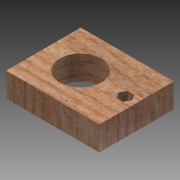
# Autodesk Inventor part: CNC-Z-axis- dremel mount
Saved by Autodesk Inventor 2015 (Build 190159000, 159)
## iProperties
Created: 2015-03-21
Part Number: CNC-Z-axis- dremel mount
Material: Generic
Document SubType Name: Modeling
Designer: Bangladesh
Density: 1 g/cm^3
Appearance: Default
Author: Bangladesh
Autodesk Inventor part; units mm, degrees
ref_plane "YZ Plane" through (0, 0, 0) normal (1, 0, 0) x (0, 1, 0)
ref_plane "XZ Plane" through (0, 0, 0) normal (0, 1, 0) x (-1, 0, 0)
ref_plane "XY Plane" through (0, 0, 0) normal (0, 0, 1) x (1, 0, 0)
sketch "Sketch1" plane through (0, 0, 0) normal (0, 1, 0) x (-1, 0, 0)
  line L0 (50, 40) -> (-50, 40)
  line L1 (-50, 40) -> (-50, -40)
  line L2 (-50, -40) -> (50, -40)
  line L3 (50, -40) -> (50, 40)
  line L4 (50, 40) -> (-50, -40) construction
  line L5 (-50, 40) -> (50, -40) construction
  point P0 (0, 0)
  dimension "d0" = 100
  dimension "d1" = 80
  constraints: 12 end point, 2 midpoint, 2 parallel, 1 horizontal, 1 perpendicular
  measures "d0" distance of L2.end L1.end
  measures "d1" distance of L1.end L0.end
extrude "Extrusion1" add sketch "Sketch1" along normal mid plane 26
sketch "Sketch2" plane through (0, 13, 0) normal (0, 1, 0) x (1, 0, 0)
  circle A0 centre (-10.17, 0) radius 22.33
  line L0 (-50, 40) -> (-50, -40) projected
  circle A1 centre (37.85, 0) radius 7.255
  line L1 (50, -40) -> (50, 40) projected
  line L2 (45.105, 0) -> (41.4775, -6.283)
  line L3 (41.4775, -6.283) -> (34.2225, -6.283)
  line L4 (34.2225, -6.283) -> (30.595, 0)
  line L5 (30.595, 0) -> (34.2225, 6.283)
  line L6 (34.2225, 6.283) -> (41.4775, 6.283)
  line L7 (41.4775, 6.283) -> (45.105, 0)
  dimension "d12" = 14.51
  dimension "d6" = 39.83
  dimension "d8" = 12.15
  constraints: 12 end point, 1 centre point, 1 coincident, 1 horizontal alignment, 15 other
  measures "d6" distance from line of L0 A0.centre
  measures "d8" distance from line of L1 point (37.85, 0)
extrude "Extrusion2" cut sketch "Sketch2" against normal blind 26 contours A0 | L2 L3 L4 L5 L6 L7
body "Solid1"
